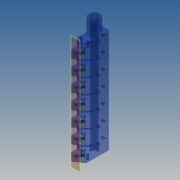
# Autodesk Inventor part: Ventilblock_3_14_M5
Saved by Autodesk Inventor 2012 (Build 160160000, 160)
## iProperties
Created: 2011-05-24
Part Number: Ventilblock_3_14_M5
Material: Edelstahl
Document SubType Name: Modeling
Designer: Neef
Mass: 556.763 g
Surface Area: 178.304 cm^2
Volume: 68.9063 cm^3
Density: 8.08 g/cm^3
Author: Neef
Autodesk Inventor part; units mm, degrees
ref_plane "YZ Plane" through (0, 0, 0) normal (1, 0, 0) x (0, 1, 0)
ref_plane "XZ Plane" through (0, 0, 0) normal (0, 1, 0) x (-1, 0, 0)
ref_plane "XY Plane" through (0, 0, 0) normal (0, 0, 1) x (1, 0, 0)
sketch "Skizze1" plane through (0, 0, 0) normal (0, 0, 1) x (1, 0, 0)
  line L0 (0, 28) -> (0, -28) projected
  line L1 (-9.1, 0) -> (9.1, 0) projected
  line L2 (-6.5, 20) -> (6.5, 20)
  line L3 (6.5, 20) -> (6.5, -20)
  line L4 (6.5, -20) -> (-6.5, -20)
  line L5 (-6.5, -20) -> (-6.5, 20)
  point P0 (0, 0)
  point P1 (0, 20)
  point P2 (-6.5, 0)
  dimension "d0" = 13
  dimension "d1" = 40
  constraints: 8 end point, 2 midpoint, 2 parallel, 2 point on line, 1 horizontal, 1 perpendicular
  measures "d0" distance of L2.start L2.end
  measures "d1" distance of L2.end L3.end
extrude "Extrusion1" add sketch "Skizze1" along normal blind 120
sketch "Skizze2" plane through (-6.5, -20, 0) normal (-1, 0, 0) x (0, 0, 1)
  line L0 (0, 40) -> (120, 40) projected
  line L1 (0, 40) -> (0, 0) projected
  point P0 (0, 20)
  point P1 (5, 34.75)
  point P2 (5, 5.25)
  dimension "d4" = 29.5
  dimension "d5" = 5.25
  dimension "d6" = 5
  dimension "d7" = 5
  measures "d4" distance of point (5, 34.75) point (5, 5.25)
  measures "d5" distance from line of L0 point (5, 34.75)
  measures "d6" distance from line of L1 point (5, 34.75)
  measures "d7" distance from line of L1 point (5, 5.25)
hole "Bohrung1" at (-6.5, 14.75, 5) at (-6.5, -14.75, 5) direction (1, 0, 0) diameter 2.459 depth 5 tip angle 118 thread size "M3x0.5" class "6H" standard "ISO Metric profile"
sketch "Skizze3" plane through (6.5, -20, 0) normal (1, 0, 0) x (0, 0, -1)
  line L0 (0, 0) -> (0, 40) projected
  line L1 (0, 40) -> (-120, 40) projected
  point P0 (0, 20)
  point P1 (-15, 34.75)
  point P2 (-15, 5.25)
  dimension "d15" = 5.25
  dimension "d16" = 29.5
  dimension "d17" = 15
  dimension "d18" = 15
  measures "d15" distance from line of L1 point (-15, 34.75)
  measures "d16" distance of point (-15, 34.75) point (-15, 5.25)
  measures "d17" distance from line of L0 point (-15, 5.25)
  measures "d18" distance from line of L0 point (-15, 34.75)
hole "Bohrung2" at (6.5, 14.75, 15) at (6.5, -14.75, 15) direction (-1, 0, 0) diameter 2.459 depth 5 tip angle 118 thread size "M3x0.5" class "6H" standard "ISO Metric profile"
sketch "Skizze4" plane through (-6.5, -20, 0) normal (-1, 0, 0) x (0, 0, 1)
  circle A0 centre (5, 34.75) radius 1.2295 projected
  point P0 (0, 20)
  point P1 (5, 26.25)
  dimension "d26" = 8.5
  measures "d26" distance of A0.centre point (5, 26.25)
hole "Bohrung3" at (-6.5, 6.25, 5) direction (1, 0, 0) diameter 1.2 depth 5 tip angle 118
sketch "Skizze5" plane through (6.5, -20, 0) normal (1, 0, 0) x (0, 0, -1)
  circle A0 centre (-15, 34.75) radius 1.2295 projected
  line L0 (0, 0) -> (0, 40) projected
  point P0 (0, 20)
  point P1 (-15, 26.25)
  dimension "d35" = 8.5
  dimension "d36" = 15
  measures "d35" distance of point (-15, 26.25) A0.centre
  measures "d36" distance from line of L0 point (-15, 26.25)
hole "Bohrung4" at (6.5, 6.25, 15) direction (-1, 0, 0) diameter 1.2 depth 5 tip angle 118
sketch "Skizze6" plane through (0, 0, 0) normal (0, 0, -1) x (-1, 0, 0)
  line L0 (6.5, 20) -> (6.5, -20) projected
  circle A0 centre (0, 6.25) radius 4
  line L1 (-12.3139, 0.15) -> (13.4676, 0.15) construction
  line L2 (-1.5, 5.65) -> (-6.5, 5.65) construction
  line L3 (-1.5, 6.85) -> (-6.5, 6.85) construction
  point P0 (0, 0)
  dimension "d44" = 8
  dimension "d45" = 6.5
  dimension "d46" = 5.5
  dimension "d48" = 0.6
  constraints: 2 end point, 1 centre point, 1 perpendicular
  measures "d44" diameter of A0
  measures "d45" distance from line of L0 A0.centre
  measures "d46" distance between parallel lines of L2 L1
  measures "d48" distance from line of L3 A0.centre
extrude "Extrusion2" cut sketch "Skizze6" against normal up to surface (120 mm away)
sketch "Skizze7" plane through (-6.5, -20, 0) normal (-1, 0, 0) x (0, 0, 1)
  circle A0 centre (5, 26.25) radius 0.6 projected
  line L0 (0, 40) -> (0, 0) projected
  point P0 (0, 20)
  point P1 (5, 18.25)
  dimension "d57" = 8
  dimension "d58" = 5
  measures "d57" distance of A0.centre point (5, 18.25)
  measures "d58" distance from line of L0 point (5, 18.25)
hole "Bohrung5" at (-6.5, -1.75, 5) direction (1, 0, 0) diameter 1.8 depth 2 tip angle 118
sketch "Skizze8" plane through (6.5, -20, 0) normal (1, 0, 0) x (0, 0, -1)
  circle A0 centre (-15, 26.25) radius 0.6 projected
  line L0 (0, 0) -> (0, 40) projected
  point P0 (0, 20)
  point P1 (-15, 18.25)
  dimension "d66" = 8
  dimension "d67" = 15
  measures "d66" distance of A0.centre point (-15, 18.25)
  measures "d67" distance from line of L0 point (-15, 18.25)
hole "Bohrung6" at (6.5, -1.75, 15) direction (-1, 0, 0) diameter 1.8 depth 2 tip angle 118
ref_plane "Arbeitsebene1" through (0, 0, 5) normal (0, 0, -1) x (-1, 0, 0)
sketch "Skizze9" plane through (0, 0, 5) normal (0, 0, -1) x (-1, 0, 0)
  line L0 (-6.5, -20) -> (6.5, -20) projected
  line L1 (6.5, -20) -> (-6.5, -10.8973)
  line L2 (-6.5, -20) -> (-6.5, 20) projected
  line L3 (-3.8396, -12.7602) -> (4.5, -0.85) construction
  line L4 (-2.3651, -13.7926) -> (5.9745, -1.8824) construction
  line L5 (-6.5, -20) -> (-6.5, 20) construction
  line L6 (-6.5, 20) -> (6.5, 20) construction
  line L7 (6.5, 20) -> (6.5, 15.9795) construction
  line L8 (6.5, 15.9795) -> (1.5, 15.9795) construction
  line L9 (1.5, 15.9795) -> (0.7612, 14.75) construction
  line L10 (0.7612, 14.75) -> (1.5, 13.5205) construction
  line L11 (1.5, 13.5205) -> (6.5, 13.5205) construction
  line L12 (6.5, 13.5205) -> (6.5, 6.85) construction
  line L13 (6.5, 6.85) -> (3.9547, 6.85) construction
  arc A0 (3.9547, 6.85) -> (3.9547, 5.65) centre (0, 6.25) ccw construction
  line L14 (3.9547, 5.65) -> (6.5, 5.65) construction
  line L15 (6.5, 5.65) -> (6.5, -0.85) construction
  line L16 (6.5, -0.85) -> (4.5, -0.85) construction
  line L17 (4.5, -0.85) -> (3.9592, -1.75) construction
  line L18 (3.9592, -1.75) -> (4.5, -2.65) construction
  line L19 (4.5, -2.65) -> (6.5, -2.65) construction
  line L20 (6.5, -2.65) -> (6.5, -13.5205) construction
  line L21 (6.5, -13.5205) -> (1.5, -13.5205) construction
  line L22 (1.5, -13.5205) -> (0.7612, -14.75) construction
  line L23 (0.7612, -14.75) -> (1.5, -15.9795) construction
  line L24 (1.5, -15.9795) -> (6.5, -15.9795) construction
  line L25 (6.5, -15.9795) -> (6.5, -20) construction
  line L26 (6.5, -20) -> (-6.5, -20) construction
  line L27 (-6.5, -20) -> (-6.5, 20) projected
  line L28 (-6.5, 20) -> (6.5, 20) projected
  line L29 (6.5, 20) -> (6.5, 15.9795) projected
  line L30 (6.5, 15.9795) -> (1.5, 15.9795) projected
  line L31 (1.5, 15.9795) -> (0.7612, 14.75) projected
  line L32 (0.7612, 14.75) -> (1.5, 13.5205) projected
  line L33 (1.5, 13.5205) -> (6.5, 13.5205) projected
  line L34 (6.5, 13.5205) -> (6.5, 6.85) projected
  line L35 (6.5, 6.85) -> (3.9547, 6.85) projected
  arc A1 (3.9547, 6.85) -> (3.9547, 5.65) centre (0, 6.25) ccw projected
  line L36 (3.9547, 5.65) -> (6.5, 5.65) projected
  line L37 (6.5, 5.65) -> (6.5, -0.85) projected
  line L38 (6.5, -0.85) -> (4.5, -0.85) projected
  line L39 (4.5, -0.85) -> (3.9592, -1.75) projected
  line L40 (3.9592, -1.75) -> (4.5, -2.65) projected
  line L41 (4.5, -2.65) -> (6.5, -2.65) projected
  line L42 (6.5, -2.65) -> (6.5, -13.5205) projected
  line L43 (6.5, -13.5205) -> (1.5, -13.5205) projected
  line L44 (1.5, -13.5205) -> (0.7612, -14.75) projected
  line L45 (0.7612, -14.75) -> (1.5, -15.9795) projected
  line L46 (1.5, -15.9795) -> (6.5, -15.9795) projected
  line L47 (6.5, -15.9795) -> (6.5, -20) projected
  line L48 (6.5, -20) -> (-6.5, -20) projected
  line L49 (4.5, -2.65) -> (4.5, -0.85) projected
  point P0 (0, 0)
  dimension "d76" = 1.8
  dimension "d77" = 35
  constraints: 8 point on line, 7 end point, 2 parallel, 1 perpendicular
  measures "d76" distance between parallel lines of L3 L4
  measures "d77" angle of L0 L1
extrude "Extrusion3" cut sketch "Skizze9" against normal mid plane 10 contours L2 L1 L0
sketch "Skizze10" plane through (-6.5, -20, 0) normal (0.5735764, -0.819152, 0) x (0.819152, 0.5735764, 0)
  ellipse E0 centre (12.1061, 5) end of major axis (12.1061, 5.9) minor radius 0.5162 projected
  point P0 (16.796, 0)
  constraints: 1 coincident, 1 other
hole "Bohrung7" at (3.4167, -13.0562, 5) direction (-0.5735764, 0.819152, 0) diameter 1.8 depth 14.3 tip angle 118
sketch "Skizze11" plane through (-6.5, -20, 0) normal (0.5735764, -0.819152, 0) x (0.819152, 0.5735764, 0)
  circle A0 centre (12.1061, 5) radius 0.9 projected
  point P0 (16.796, 0)
  constraints: 1 coincident
hole "Bohrung8" at (3.4167, -13.0562, 5) direction (-0.5735764, 0.819152, 0) diameter 4.134 depth 4 tip angle 118 thread size "M5x0.8" class "6H" standard "ISO Metric profile"
ref_plane "Arbeitsebene2" through (0, 0, 15) normal (0, 0, -1) x (-1, 0, 0)
sketch "Skizze12" plane through (0, 0, 15) normal (0, 0, -1) x (-1, 0, 0)
  line L0 (-0.7612, 14.75) -> (-1.5, 15.9795) projected
  line L1 (-1.5, 15.9795) -> (-6.5, 15.9795) projected
  line L2 (-6.5, 15.9795) -> (-6.5, 20) projected
  line L3 (-6.5, 20) -> (6.5, 20) projected
  line L4 (6.5, 20) -> (6.5, -20) projected
  line L5 (6.5, -20) -> (-6.5, -20) projected
  line L6 (-6.5, -20) -> (-6.5, -15.9795) projected
  line L7 (-6.5, -15.9795) -> (-1.5, -15.9795) projected
  line L8 (-1.5, -15.9795) -> (-0.7612, -14.75) projected
  line L9 (-0.7612, -14.75) -> (-1.5, -13.5205) projected
  line L10 (-1.5, -13.5205) -> (-6.5, -13.5205) projected
  line L11 (-6.5, -13.5205) -> (-6.5, -2.65) projected
  line L12 (-6.5, -2.65) -> (-4.5, -2.65) projected
  line L13 (-4.5, -2.65) -> (-3.9592, -1.75) projected
  line L14 (-3.9592, -1.75) -> (-4.5, -0.85) projected
  line L15 (-4.5, -0.85) -> (-6.5, -0.85) projected
  line L16 (-6.5, -0.85) -> (-6.5, 5.65) projected
  line L17 (-6.5, 5.65) -> (-3.9547, 5.65) projected
  arc A0 (-3.9547, 5.65) -> (-3.9547, 6.85) centre (0, 6.25) ccw projected
  line L18 (-3.9547, 6.85) -> (-6.5, 6.85) projected
  line L19 (-6.5, 6.85) -> (-6.5, 13.5205) projected
  line L20 (-6.5, 13.5205) -> (-1.5, 13.5205) projected
  line L21 (-1.5, 13.5205) -> (-0.7612, 14.75) projected
  line L22 (-6.5, -20) -> (6.5, -10.8973)
  line L23 (6.5, 20) -> (6.5, -20) projected
  point P0 (0, 0)
  dimension "d95" = 35
  constraints: 2 end point, 1 point on line
  measures "d95" angle of L5 L22
extrude "Extrusion4" cut sketch "Skizze12" against normal mid plane 10 contours L4 L5 L22
sketch "Skizze13" plane through (-6.5, -10.8973, 10) normal (-0.5735764, -0.819152, 0) x (0.819152, -0.5735764, 0)
  ellipse E0 centre (3.764, 5) end of major axis (3.764, 4.1) minor radius 0.5162 projected
  point P0 (-0.9259, -10)
  constraints: 1 coincident, 1 other
hole "Bohrung9" at (-3.4167, -13.0562, 15) direction (0.5735764, 0.819152, 0) diameter 1.8 depth 14.3 tip angle 118
sketch "Skizze14" plane through (-6.5, -10.8973, 10) normal (-0.5735764, -0.819152, 0) x (0.819152, -0.5735764, 0)
  circle A0 centre (3.764, 5) radius 0.9 projected
  point P0 (-0.9259, -10)
  point P1 (3.764, 5)
  constraints: 1 coincident
hole "Bohrung10" at (-3.4167, -13.0562, 15) direction (0.5735764, 0.819152, 0) diameter 4.134 depth 4 tip angle 118 thread size "M5x0.8" class "6H" standard "ISO Metric profile"
pattern_linear "Rechteckige Anordnung3" count 5 spacing 20 along (0, 0, 1) of "Bohrung1", "Bohrung2", "Bohrung3", "Bohrung4", "Bohrung5", "Bohrung6", "Extrusion3", "Bohrung7", "Bohrung8", "Extrusion4", "Bohrung9", "Bohrung10"
sketch "Skizze15" plane through (0, 0, 120) normal (0, 0, 1) x (1, 0, 0)
  circle A0 centre (0, 6.25) radius 4 projected
  point P0 (0, 0)
  constraints: 1 coincident
hole "Bohrung11" at (0, 6.25, 120) direction (0, 0, -1) diameter 8.566 depth 10 tip angle 118 thread size "G9.728x0.907" designation "G 1/8" standard "ISO Pipe Threads"
ref_plane "Arbeitsebene3" through (0, 6.25, 0) normal (0, -1, 0) x (0, 0, 1)
sketch "Skizze18" plane through (0, 0, 120) normal (0, 0, 1) x (1, 0, 0)
  circle A0 centre (0, 6.25) radius 4.283 projected
  line L0 (-6.5, 20) -> (6.5, 20)
  line L1 (6.5, -20) -> (-6.5, -20)
  line L2 (6.5, 20) -> (6.5, 9.9917)
  line L3 (6.5, 2.5083) -> (6.5, -20)
  line L4 (-6.5, -20) -> (-6.5, 2.5083)
  line L5 (-6.5, 9.9917) -> (-6.5, 20)
  arc A1 (6.5, 9.9917) -> (-6.5, 9.9917) centre (0, 6.25) ccw
  arc A2 (-6.5, 2.5083) -> (6.5, 2.5083) centre (0, 6.25) ccw
  point P0 (0, 0)
  constraints: 12 end point, 5 parallel, 4 point on circle, 2 centre point, 2 perpendicular, 1 coincident, 1 horizontal
extrude "Extrusion6" cut sketch "Skizze18" against normal blind 20 contours L0 L2 A1 L5 | L1 L4 A2 L3
fillet "Rundung1" radius 1 16 edges at (-6.5, 20, 50) (6.5, 20, 50) (-6.5, -20, 5) (6.5, -20, 15) (-6.5, -20, 25) (6.5, -20, 35) (-6.5, -20, 45) (6.5, -20, 55) (-6.5, -20, 65) (6.5, -20, 75) (-6.5, -20, 85) (6.5, -20, 95) (0, 13.75, 120) (-6.5, 6.25, 120) (0, -1.25, 120) (6.5, 6.25, 120)
sketch "Skizze19" plane through (0, 0, 100) normal (0, 0, 1) x (1, 0, 0)
  circle A0 centre (-4.5, -7.15) radius 1.1 projected
  circle A1 centre (4.5, -7.15) radius 1.1 projected
  point P0 (0, 0)
  constraints: 2 coincident
hole "Bohrung13" at (-4.5, -7.15, 100) at (4.5, -7.15, 100) direction (0, 0, -1) diameter 2.459 depth 8 tip angle 118 thread size "M3x0.5" class "6H" standard "ISO Metric profile"
sketch "Skizze21" plane through (6.5, -10.8973, 10) normal (1, 0, 0) x (0, 0, -1)
  circle A0 centre (5, 25.6473) radius 1.2295 projected
  circle A1 centre (5, -3.8527) radius 1.2295 projected
  line L0 (10, -8.1817) -> (0, -8.1817) projected
  line L1 (10, 30.8973) -> (-90, 30.8973) projected
  line L2 (5, 30.8973) -> (10, 30.8973)
  line L3 (10, 30.8973) -> (10, -8.1817)
  line L4 (10, -8.1817) -> (5, -8.1817)
  line L5 (5, -8.1817) -> (5, 30.8973)
  constraints: 8 end point, 2 parallel, 1 horizontal, 1 perpendicular, 1 point on line
extrude "Extrusion7" cut sketch "Skizze21" against normal up to surface (13 mm away) contours A0 L5 | A0 L5 L1 L3 L0 A1 | A1 L5 picked at (5.4379, 25.9677) picked at (5.4908, -3.7718)
mirror "Spiegeln1" about plane through (6.5, 20, 5) normal (0, 0, -1)
sketch "Skizze22" plane through (6.5, -10.8973, 90) normal (1, 0, 0) x (0, 0, -1)
  circle A0 centre (175, 25.6473) radius 1.2295 projected
  circle A1 centre (175, -3.8527) radius 1.2295 projected
  circle A2 centre (175, 17.1473) radius 0.6 projected
  circle A3 centre (135, 25.6473) radius 1.2295 projected
  circle A4 centre (135, -3.8527) radius 1.2295 projected
  circle A5 centre (135, 17.1473) radius 0.6 projected
  circle A6 centre (135, 9.1473) radius 0.9 projected
  circle A7 centre (155, 9.1473) radius 0.9 projected
  circle A8 centre (175, 9.1473) radius 0.9 projected
  circle A9 centre (155, 17.1473) radius 0.6 projected
  circle A10 centre (155, -3.8527) radius 1.2295 projected
  circle A11 centre (155, 25.6473) radius 1.2295 projected
  line L0 (140, -8.1817) -> (130, -8.1817) projected
  line L1 (130, -7.1817) -> (130, -8.1817) projected
  line L2 (180, 30.8973) -> (-10, 30.8973) projected
  line L3 (130, -8.1817) -> (200, -8.1817)
  line L4 (200, -8.1817) -> (200, 30.8973)
  line L5 (200, 30.8973) -> (130, 30.8973)
  line L6 (130, 30.8973) -> (130, -8.1817)
  point P0 (130, -8.0009)
  constraints: 8 end point, 2 parallel, 1 horizontal, 1 perpendicular
extrude "Extrusion8" cut sketch "Skizze22" against normal up to surface (13 mm away) contours A0 | A1 | A2 | A3 | A4 | A5 | A6 | A7 | A8 | A9 | A10 | A11 | L0 L1 L6 L2 L5 L4 L3
sketch "Skizze23" plane through (0, 6.25, 0) normal (0, -1, 0) x (0, 0, 1)
  line L0 (94.4, -6.5) -> (75.6, -6.5) projected
  line L1 (75.6, -6.5) -> (75.6, -4) projected
  line L2 (75.6, -4) -> (94.4, -4) projected
  line L3 (94.4, -4) -> (94.4, -6.5) projected
  line L4 (74.4, -6.5) -> (55.6, -6.5) projected
  line L5 (55.6, -6.5) -> (55.6, -4) projected
  line L6 (55.6, -4) -> (74.4, -4) projected
  line L7 (74.4, -4) -> (74.4, -6.5) projected
  line L8 (54.4, -6.5) -> (35.6, -6.5) projected
  line L9 (35.6, -6.5) -> (35.6, -4) projected
  line L10 (35.6, -4) -> (54.4, -4) projected
  line L11 (54.4, -4) -> (54.4, -6.5) projected
  line L12 (34.4, -6.5) -> (15.6, -6.5) projected
  line L13 (15.6, -6.5) -> (15.6, -4) projected
  line L14 (15.6, -4) -> (34.4, -4) projected
  line L15 (34.4, -4) -> (34.4, -6.5) projected
  line L16 (14.4, -6.5) -> (-4.4, -6.5) projected
  line L17 (-4.4, -6.5) -> (-4.4, -4) projected
  line L18 (-4.4, -4) -> (14.4, -4) projected
  line L19 (14.4, -4) -> (14.4, -6.5) projected
  line L20 (-5.6, -6.5) -> (-24.4, -6.5) projected
  line L21 (-24.4, -6.5) -> (-24.4, -4) projected
  line L22 (-24.4, -4) -> (-5.6, -4) projected
  line L23 (-5.6, -4) -> (-5.6, -6.5) projected
  line L24 (-25.6, -6.5) -> (-40, -6.5) projected
  line L25 (-40, -6.5) -> (-40, -4) projected
  line L26 (-40, -4) -> (-25.6, -4) projected
  line L27 (-25.6, -4) -> (-25.6, -6.5) projected
  line L28 (-35.6, 6.5) -> (-35.6, 4) projected
  line L29 (-35.6, 4) -> (-40, 4) projected
  line L30 (-40, 4) -> (-40, 6.5) projected
  line L31 (-40, 6.5) -> (-35.6, 6.5) projected
  line L32 (-34.4, 4) -> (-34.4, 6.5) projected
  line L33 (-34.4, 6.5) -> (-15.6, 6.5) projected
  line L34 (-15.6, 6.5) -> (-15.6, 4) projected
  line L35 (-15.6, 4) -> (-34.4, 4) projected
  line L36 (5.6, 4) -> (5.6, 6.5) projected
  line L37 (5.6, 6.5) -> (24.4, 6.5) projected
  line L38 (24.4, 6.5) -> (24.4, 4) projected
  line L39 (24.4, 4) -> (5.6, 4) projected
  line L40 (4.4, 6.5) -> (4.4, 4) projected
  line L41 (4.4, 4) -> (-14.4, 4) projected
  line L42 (-14.4, 4) -> (-14.4, 6.5) projected
  line L43 (-14.4, 6.5) -> (4.4, 6.5) projected
  line L44 (25.6, 6.5) -> (44.4, 6.5) projected
  line L45 (44.4, 6.5) -> (44.4, 4) projected
  line L46 (44.4, 4) -> (25.6, 4) projected
  line L47 (25.6, 4) -> (25.6, 6.5) projected
  line L48 (45.6, 6.5) -> (64.4, 6.5) projected
  line L49 (64.4, 6.5) -> (64.4, 4) projected
  line L50 (64.4, 4) -> (45.6, 4) projected
  line L51 (45.6, 4) -> (45.6, 6.5) projected
  line L52 (65.6, 6.5) -> (84.4, 6.5) projected
  line L53 (84.4, 6.5) -> (84.4, 4) projected
  line L54 (84.4, 4) -> (65.6, 4) projected
  line L55 (65.6, 4) -> (65.6, 6.5) projected
  line L56 (109.83, -4) -> (110, -4.283) projected
  line L57 (110, -4.283) -> (120, -4.283) projected
  line L58 (120, -4.283) -> (120, -5.5) projected
  arc A0 (119, -6.5) -> (120, -5.5) centre (119, -5.5) ccw projected
  line L59 (119, -6.5) -> (95.6, -6.5) projected
  line L60 (95.6, -6.5) -> (95.6, -4) projected
  line L61 (95.6, -4) -> (109.83, -4) projected
  line L62 (110, 4.283) -> (109.83, 4) projected
  line L63 (109.83, 4) -> (85.6, 4) projected
  line L64 (85.6, 4) -> (85.6, 6.5) projected
  line L65 (85.6, 6.5) -> (119, 6.5) projected
  arc A1 (120, 5.5) -> (119, 6.5) centre (119, 5.5) ccw projected
  line L66 (120, 5.5) -> (120, 4.283) projected
  line L67 (120, 4.283) -> (110, 4.283) projected
  line L68 (-38.5194, 4) -> (-39.3064, 2.1)
  line L69 (-39.3064, 2.1) -> (-40, 2.1)
  line L70 (-40, -5.5) -> (-40, 5.5) projected
  line L71 (-40.5027, 0) -> (-33.0365, 0) construction
  line L72 (-40, -4) -> (109.83, -4) construction
  line L73 (-40, 2.1) -> (-40, 4)
  line L74 (-40, 4.9264) -> (-40, -6.5) projected
  line L75 (-38.5194, 4) -> (-40, 4)
  dimension "d159" = 67.5
  dimension "d160" = 4
  dimension "d161" = 2.1
  constraints: 10 end point, 2 collinear, 2 point on line, 1 horizontal, 1 parallel, 1 other
  measures "d159" angle of L69 L68
  measures "d160" distance between parallel lines of L29 L71
  measures "d161" distance between parallel lines of L69 L71
revolve "Umdrehung2" add sketch "Skizze23" angle 360 about axis through (0, 6.25, -40.5027) along (0, 0, 1) contours L68 L69 L70 L29
sketch "Skizze24" plane through (5.5, 20, -40) normal (0, 0, -1) x (-1, 0, 0)
  circle A0 centre (5.5, -13.75) radius 2.1 projected
  circle A1 centre (5.5, -13.75) radius 4
  dimension "d163" = 8
  constraints: 1 centre point, 1 coincident
  measures "d163" diameter of A1
extrude "Extrusion9" add sketch "Skizze24" along normal blind 12
thread "Gewinde1" size "M5x0.8" class "6H" standard "ANSI Metric M Profile" length 8
ref_plane "Arbeitsebene4" through (0, 0, 30) normal (0, 0, 1) x (1, 0, 0)
mirror "Spiegeln2" about plane through (0, 0, 30) normal (0, 0, 1) of "Bohrung13"
sketch "Skizze25" plane through (0, 0, 120) normal (0, 0, 1) x (1, 0, 0)
  circle A0 centre (0, 6.25) radius 4.283 projected
  line L0 (5.5, 9.7141) -> (5.5, 2.7859) projected
  arc A1 (5.5, 9.7141) -> (-5.5, 9.7141) centre (0, 6.25) ccw projected
  line L1 (-5.5, 2.7859) -> (-5.5, 9.7141) projected
  arc A2 (-5.5, 2.7859) -> (5.5, 2.7859) centre (0, 6.25) ccw projected
  arc A3 (-6.5, -18.079) -> (-4.9264, -18.8982) centre (-5.5, -18.079) ccw projected
  arc A4 (4.9264, -18.8982) -> (6.5, -18.079) centre (5.5, -18.079) ccw projected
  line L2 (-1.3215, -19.079) -> (5.4851, -19.079)
  line L3 (-5.5, 20) -> (5.5, 20) projected
  point P0 (0, 0)
  constraints: 2 end point, 1 parallel, 1 tangent
ref_plane "Arbeitsebene5" through (-5.5, -19.1, 100) normal (0, 1, 0) x (1, 0, 0)
move faces "Fläche verschieben1" translate (0, 0, 12) faces at (-3.3279, 5.9309, -52)
sketch "Skizze26" plane through (5.5, 20, -40) normal (0, 0, -1) x (-1, 0, 0)
  circle A0 centre (5.5, -13.75) radius 2.1 projected
  circle A1 centre (5.5, -13.75) radius 4.4
  point P0 (5.5, -20)
  dimension "d173" = 8.8
  constraints: 1 centre point, 1 coincident
  measures "d173" diameter of A1
extrude "Extrusion10" cut sketch "Skizze26" against normal blind 8
thread "Gewinde2" size "G9.728x0.907" designation "G 1/8" standard "ISO Pipe Threads" full length
equation "\"d7\" = d6"
equation "\"d18\" = d17"
